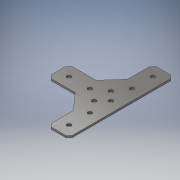
# Autodesk Inventor part: 1in tbracket for alu extrusions
Saved by Autodesk Inventor 2017 (Build 210142000, 142)
## iProperties
Created: 2016-10-02
Part Number: 1in tbracket for alu extrusions
Material: Steel, Alloy
Document SubType Name: Modeling
Designer: Aditya
Density: 7.73 g/cm^3
Appearance: Semi-Polished
Author: Aditya
Autodesk Inventor part; units mm, degrees
ref_plane "YZ Plane" through (0, 0, 0) normal (1, 0, 0) x (0, 1, 0)
ref_plane "XZ Plane" through (0, 0, 0) normal (0, 1, 0) x (-1, 0, 0)
ref_plane "XY Plane" through (0, 0, 0) normal (0, 0, 1) x (1, 0, 0)
sketch "Sketch1" plane through (0, 0, 0) normal (0, 1, 0) x (-1, 0, 0)
  line L0 (25.4, -30.48) -> (43.18, -50.8)
  line L1 (25.4, -96.52) -> (43.18, -76.2)
  line L2 (3.81, 0) -> (0, -3.81)
  line L3 (0, -123.19) -> (3.81, -127)
  line L4 (25.4, -123.19) -> (21.59, -127)
  line L5 (25.4, -3.81) -> (21.59, 0)
  line L6 (72.39, -50.8) -> (76.2, -54.61)
  line L7 (76.2, -72.39) -> (72.39, -76.2)
  line L8 (25.4, -3.81) -> (25.4, -30.48)
  line L9 (43.18, -50.8) -> (72.39, -50.8)
  line L10 (76.2, -54.61) -> (76.2, -72.39)
  line L11 (72.39, -76.2) -> (43.18, -76.2)
  line L12 (25.4, -96.52) -> (25.4, -123.19)
  line L13 (21.59, -127) -> (3.81, -127)
  line L14 (0, -123.19) -> (0, -3.81)
  line L15 (3.81, 0) -> (21.59, 0)
  circle A0 centre (12.7, -12.7) radius 2.54
  circle A1 centre (12.7, -38.1) radius 2.54
  circle A2 centre (12.7, -63.5) radius 2.54
  circle A3 centre (12.7, -88.9) radius 2.54
  circle A4 centre (12.7, -114.3) radius 2.54
  circle A5 centre (63.5, -63.5) radius 2.54
  circle A6 centre (38.1, -63.5) radius 2.54
  circle A7 centre (22.86, -53.34) radius 2.54
  circle A8 centre (22.86, -73.66) radius 2.54
  point P0 (0, 0)
  constraints: 32 end point, 9 centre point, 7 perpendicular, 1 vertical
extrude "Extrusion1" add sketch "Sketch1" along normal blind 2.54
body "Solid1"
